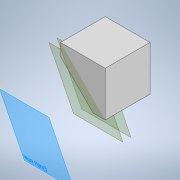
# Autodesk Inventor part: joint
Saved by Autodesk Inventor 2022 (Build 260153000, 153)
## iProperties
Created: 2022-06-09
Part Number: joint
Material: Generic
Document SubType Name: Modeling
Designer: logic
Density: 1 g/cm^3
Appearance: Default
Author: logic
Autodesk Inventor part; units mm, degrees
ref_plane "YZ Plane" through (0, 0, 0) normal (1, 0, 0) x (0, 1, 0)
ref_plane "XZ Plane" through (0, 0, 0) normal (0, 1, 0) x (-1, 0, 0)
ref_plane "XY Plane" through (0, 0, 0) normal (0, 0, 1) x (1, 0, 0)
sketch "Sketch11" plane through (0, 0, 0) normal (1, 0, 0) x (0, 1, 0)
  line L0 (11, -11) -> (-11, -11)
  line L1 (-11, -11) -> (-11, 11)
  line L2 (-11, 11) -> (11, 11)
  line L3 (11, 11) -> (11, -11)
  line L4 (16, -16) -> (-16, -16)
  line L5 (-16, -16) -> (-16, 16)
  line L6 (-16, 16) -> (16, 16)
  line L7 (16, 16) -> (16, -16)
  point P0 (0, 0)
  dimension "d39" = 22
  dimension "d40" = 22
  dimension "d41" = 11
  dimension "d42" = 11
  dimension "d43" = 5
  dimension "d44" = 5
  dimension "d45" = 5
  dimension "d46" = 5
  constraints: 16 end point, 4 parallel, 2 horizontal, 2 perpendicular
  measures "d39" distance of L1.end L2.end
  measures "d40" distance of L0.end L1.end
  measures "d41" distance from line of point (0, 0) L3
  measures "d42" distance from line of L2 point (0, 0)
  measures "d43" distance between parallel lines of L3 L7
  measures "d44" distance between parallel lines of L6 L2
  measures "d45" distance between parallel lines of L5 L1
  measures "d46" distance between parallel lines of L4 L0
extrude "Extrusion8" add sketch "Sketch11" against normal blind 32 contours L0 L1 L2 L3 | L4 L5 L6 L7
ref_plane "Work Plane4" through (-34.8868, 13.1132, 18.8868) normal (-0.5773503, -0.5773503, 0.5773503) x (0, -0.7071068, -0.7071068)
ref_plane "Work Plane3" through (-32, 16, 16) normal (-0.5773503, -0.5773503, 0.5773503) x (0, -0.7071068, -0.7071068)
sketch "Sketch14" plane through (-34.8868, 13.1132, 18.8868) normal (-0.5773503, -0.5773503, 0.5773503) x (0, -0.7071068, -0.7071068)
  line L0 (45.2548, 0) -> (22.6274, 13.0639) projected
  line L1 (4.8978, 38.1971) -> (41.7061, 38.1971)
  line L2 (41.7061, 38.1971) -> (41.7061, 2.0489)
  line L3 (41.7061, 2.0489) -> (4.8978, 2.0489)
  line L4 (4.8978, 2.0489) -> (4.8978, 38.1971)
  point P0 (22.6274, 26.1279)
  constraints: 8 end point, 2 parallel, 1 horizontal, 1 perpendicular, 1 point on line
extrude "Extrusion11" cut sketch "Sketch14" along normal blind 29.75
sketch "Sketch16" plane through (0, 0, 0) normal (1, 0, 0) x (0, 0, -1)
  line L0 (-11, 11) -> (11, 11)
  line L1 (11, 11) -> (11, -11)
  line L2 (11, -11) -> (-11, -11)
  line L3 (-11, -11) -> (-11, 11)
  line L4 (-16, 16) -> (16, 16)
  line L5 (16, 16) -> (16, -16)
  line L6 (16, -16) -> (-16, -16)
  line L7 (-16, -16) -> (-16, 16)
  point P0 (0, 0)
  dimension "d60" = 22
  dimension "d61" = 22
  dimension "d62" = 11
  dimension "d63" = 11
  constraints: 16 end point, 4 parallel, 2 coincident, 2 horizontal, 2 perpendicular
  measures "d60" distance of L1.end L2.end
  measures "d61" distance of L0.end L1.end
  measures "d62" distance from line of L2 point (0, 0)
  measures "d63" distance from line of L1 point (0, 0)
extrude "Extrusion12" add sketch "Sketch16" along normal blind 50
sketch "Sketch17" plane through (-32, 16, 16) normal (0, 1, 0) x (1, 0, 0)
  line L0 (32, 32) -> (0, 32)
  line L1 (0, 32) -> (0, 0)
  line L2 (0, 0) -> (32, 0)
  line L3 (32, 0) -> (32, 32)
  line L4 (0, 32) -> (82, 32) projected
  line L5 (27, 27) -> (5, 27)
  line L6 (5, 27) -> (5, 5)
  line L7 (5, 5) -> (27, 5)
  line L8 (27, 5) -> (27, 27)
  point P0 (32, 16)
  dimension "d66" = 22
  dimension "d67" = 22
  dimension "d68" = 5
  dimension "d69" = 5
  constraints: 16 end point, 4 parallel, 2 horizontal, 2 perpendicular, 1 coincident, 1 midpoint, 1 point on line
  measures "d66" distance of L7.end L6.end
  measures "d67" distance of L6.end L5.end
  measures "d68" distance between parallel lines of L2 L7
  measures "d69" distance between parallel lines of L1 L6
extrude "Extrusion13" add sketch "Sketch17" along normal blind 50
sketch "Sketch18" plane through (50, -16, -16) normal (0, 0, -1) x (-1, 0, 0)
  line L0 (50, 32) -> (82, 32)
  line L1 (82, 32) -> (82, 0)
  line L2 (82, 0) -> (50, 0)
  line L3 (50, 0) -> (50, 32)
  line L4 (55, 27) -> (77, 27)
  line L5 (77, 27) -> (77, 5)
  line L6 (77, 5) -> (55, 5)
  line L7 (55, 5) -> (55, 27)
  point P0 (50, 16)
  dimension "d72" = 22
  dimension "d73" = 22
  dimension "d74" = 5
  dimension "d75" = 5
  constraints: 16 end point, 4 parallel, 2 coincident, 2 horizontal, 2 perpendicular
  measures "d72" distance of L5.end L6.end
  measures "d73" distance of L4.end L5.end
  measures "d74" distance between parallel lines of L4 L0
  measures "d75" distance between parallel lines of L1 L5
extrude "Extrusion14" add sketch "Sketch18" along normal blind 50
fillet "Fillet1" radius 5 6 edges at (-32, 36.6716, 16) (-20.3284, -4.3284, 16) (-32, -4.3284, 4.3284) (-20.3284, -16, 4.3284) (20.6716, -16, 16) (-32, -16, -36.6716)
fillet "Fillet2" radius 5 12 edges at (0, 41, -16) (25, 16, -16) (0, 16, -41) (0, 0, -16) (0, -16, -41) (25, -16, -16) (0, 16, 0) (-16, 16, -16) (-32, 41, -16) (-32, 16, -41) (0, 41, 16) (25, 16, 16)
body "Solid3"
